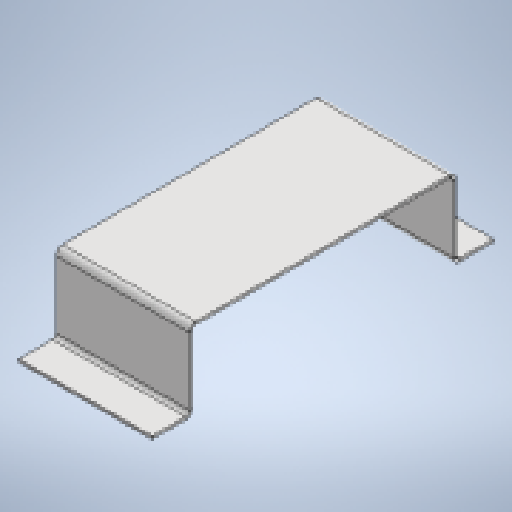
# Autodesk Inventor part: BSH pollar 5
Saved by Autodesk Inventor 2025.1 (Build 291241020, 241B)
## iProperties
Created: 2024-09-23
Part Number: BSH pollar 5
Material: Stainless Steel
Document SubType Name: Sheet Metal
Designer: user
Density: 8 g/cm^3
Flat Pattern Width: 14 cm
Flat Pattern Length: 38.4808 cm
Flat Pattern Area: 538.731 cm^2
Sheet Metal Rule: AISI304 2mm Die16
Sheet Metal Width: 140.000 mm
Sheet Metal Length: 384.808 mm
Sheet Metal Area: 53873.115 mm^2
Appearance: Default
Author: user
Autodesk Inventor part; units mm, degrees
ref_plane "YZ Plane" through (0, 0, 0) normal (1, 0, 0) x (0, 1, 0)
ref_plane "XZ Plane" through (0, 0, 0) normal (0, 1, 0) x (-1, 0, 0)
ref_plane "XY Plane" through (0, 0, 0) normal (0, 0, 1) x (1, 0, 0)
sketch "Sketch1" plane through (0, 0, 0) normal (0, 0, 1) x (1, 0, 0)
  line L0 (-70, -135) -> (70, -135)
  line L1 (70, -135) -> (70, 135)
  line L2 (70, 135) -> (-70, 135)
  line L3 (-70, 135) -> (-70, -135)
  line L4 (-70, -135) -> (70, 135) construction
  line L5 (70, -135) -> (-70, 135) construction
  point P0 (0, 0)
  dimension "d0" = 140
  dimension "d1" = 270
  measures "d0" distance of L2.end L1.end
  measures "d1" distance of L1.end L0.end
extrude "Plate1" add sketch "Sketch1" along normal blind 2
sketch "Sketch3" plane through (70, 133, 2) normal (0, 1, 0) x (-1, 0, 0)
  line L0 (140, 0) -> (0, 0)
  line L1 (0, 0) -> (0, -50)
  line L2 (0, -50) -> (140, -50)
  line L3 (140, -50) -> (140, 0)
  constraints: 6 end point, 1 horizontal, 1 perpendicular, 1 vertical
edge flange "Flange1" height 50 angle 90 thickness 2 bend radius 2.75 thickness toward (0, 1, 0) relief round relief width 2 relief depth 1 corner gap 2.75 corner form 0 edges at (0, 135, 0) (0, -135, 0) wall of the first edge with corners at (-70, 133, 2) (70, 133, 2) (70, 133, -48) (-70, 133, -48)
bend "Bend1"
corner "Corner1"
sketch "Sketch4" plane through (-70, 133, -46) normal (0, 0, -1) x (-1, 0, 0)
  line L0 (-140, 0) -> (0, 0)
  line L1 (0, 0) -> (0, 15)
  line L2 (0, 15) -> (-140, 15)
  line L3 (-140, 15) -> (-140, 0)
  constraints: 6 end point, 1 horizontal, 1 perpendicular, 1 vertical
edge flange "Flange2" height 15 angle 90 thickness 2 bend radius 2.75 thickness toward (0, 0, -1) relief round relief width 2 relief depth 1 corner gap 2.75 corner form 0 edges at (0, 135, -48) (0, -135, -48) wall of the first edge with corners at (70, 133, -46) (-70, 133, -46) (-70, 148, -46) (70, 148, -46)
bend "Bend2"
corner "Corner2"
equation "\"d2\" = Thickness"
equation "\"d6\" = BendReliefWidth"
equation "\"d7\" = BendReliefDepth"
equation "\"d8\" = MinimumRemnant"
equation "\"d9\" = TransitionRadius"
equation "\"d12\" = BendRadius"
equation "\"d13\" = CornerReliefSize"
equation "\"d14\" = GapSize"
equation "\"d15\" = JacobiRadiusSize"
equation "\"d16\" = BendReliefWidth"
equation "\"d17\" = BendReliefDepth"
equation "\"d18\" = MinimumRemnant"
equation "\"d19\" = TransitionRadius"
equation "\"d22\" = BendRadius"
equation "\"d23\" = CornerReliefSize"
equation "\"d24\" = GapSize"
equation "\"d25\" = JacobiRadiusSize"
equation "\"BendReliefWidth\" = Thickness"
equation "\"BendReliefDepth\" = 0.5 * Thickness"
equation "\"CornerReliefSize\" = 4 * Thickness"
equation "\"MinimumRemnant\" = 2 * Thickness"
equation "\"TransitionRadius\" = BendRadius"
equation "\"JacobiRadiusSize\" = BendRadius"
equation "\"GapSize\" = Thickness"
equation "\"Thickness\" = 2"
equation "\"BendRadius\" = 2.75"
body "Solid1"
